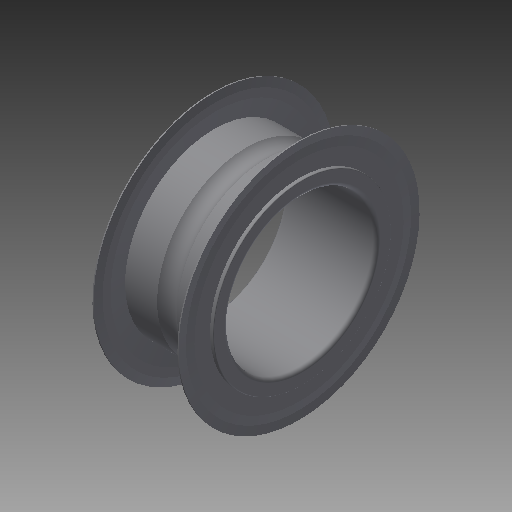
# Autodesk Inventor part: W 627/4-2Z_PART1
Saved by Autodesk Inventor 2018.3 (Build 223284000, 284)
## iProperties
Category: PARTsolutions
Company: SKF
Created: 2018-07-21
Part Number: W 627/4-2Z_PART1
Material: Generic
Catalog Web Link: www.cadenas.de
Description: -Deep groove ball bearings, stainless steel, single row
Vendor: SKF
Document SubType Name: Modeling
Designer: psadmin
Manufacturer: SKF
Mass: 0.0145905 g
Surface Area: 1.40149 cm^2
Volume: 0.0145905 cm^3
Density: 1 g/cm^3
Appearance: PSOLRGB-175-175-175
PSOL_IDENT_0: {$CADENAS_DATA\23d-libs\skf\bearings_units_and_housings\ball_bearings\deep_groove_ball_bearings\deep
PSOL_IDENT_1: _groove_ball_bearings_stainless_steel\bb1_004_104.prj},199 {VTYP=3D},{NB=W 627/4-2Z_PART1},{LINA=W 6
PSOL_IDENT_2: 27/4-2Z_PART1},{NN=BB1_004_104_PART1},{NOPRJ=TRUE},{DATE=13.07.2018 14:28:03},{GEOMDATE=26.07.2017 1
PSOL_IDENT_3: 2:34:56},{VERSION=},{LINEID=77220},{WBVAR=},{WBNUMERIC=}  {NB=W 627/4-2Z_PART1},{LINA=W 627/4-2Z_PAR
PSOL_IDENT_4: T1},{KT=DUMMY},{PRODUCTID=},{DESIGNATION=W 627/4-2Z},{DD=4.000},{D=7.000},{B=2.500},{DD1=4.800},{DD2=
PSOL_IDENT_5: MIN},{D1=6.000},{D2=6.500},{R12A=0.100},{LOAD1=0.143},{LOAD2=0.053},{LOAD3=0.002},{SPEED1=75000},{SP
PSOL_IDENT_6: EED2=},{MASS=0.000},{PITCH=5.400},{DW=0.800},{Z=11.000},{II=1.000},{TYPEID=MIN},{YALG=2.4},{HALG=0.4
PSOL_IDENT_7: },{HELP=0.5},{HELP2=0.25},{YALG1=3},{HALG1=0.5},{TAXONOMY=2},{DESIGN=dgbbw2z},{MAPPING=BCZ50,DESIGNA
PSOL_IDENT_8: TION|IRD01,DD|ORD10,D|BCW30,B|IRD30,DD1|ORD30,D1|ORD43,D2|IRD43,DD2|ORR20,R12A|BCC02,LOAD1|BCC16,LOA
PSOL_IDENT_9: D2|BCC12,LOAD3|BCC45,SPEED1|BCM01,MASS|BCD50,PITCH|RBD10,DW|BCN81,Z|BCN80,II},{DESIGNLIST=dgbbw2z,dg
PSOL_IDENT_10: bbw,dgbbw2rs},{SH=2.4},{SORT=DD},{RHELP=0.1},{PIM=W 627/4-2Z},{R12=0.1},{HIDE=MIN}
NT: Deep groove ball bearings, stainless steel, single row
NB: W 627/4-2Z_PART1
NBSYN: $DESIGNATION._PART1
LINA: W 627/4-2Z_PART1
SUPPLIER: SKF
ARTICLENO: W 627/4-2Z_PART1
BOMINFO: W 627/4-2Z_PART1
CREATOR: CADENAS GmbH
Title: W 627/4-2Z_PART1
Author: Cadenas PARTsolutions
Comments: Deep groove ball bearings, stainless steel, single row
Autodesk Inventor part; units mm, degrees
ref_plane "YZ Plane" through (0, 0, 0) normal (1, 0, 0) x (0, 1, 0)
ref_plane "XZ Plane" through (0, 0, 0) normal (0, 1, 0) x (-1, 0, 0)
ref_plane "XY Plane" through (0, 0, 0) normal (0, 0, 1) x (1, 0, 0)
sketch "Sketch_6" plane through (0, 0, 0) normal (0, 0, 1) x (1, 0, 0)
  line L0 (50, 0) -> (-50, 0)
  line L1 (0, 2.38) -> (0, 2.1)
  arc A0 (0, 2.1) -> (0.1, 2) centre (0.1, 2.1) ccw
  line L2 (0.1, 2) -> (2.4, 2)
  arc A1 (2.4, 2) -> (2.5, 2.1) centre (2.4, 2.1) ccw
  line L3 (2.5, 2.1) -> (2.5, 2.38)
  arc A2 (2.5, 2.38) -> (2.48, 2.4) centre (2.48, 2.38) ccw
  line L4 (2.48, 2.4) -> (1.5146, 2.4)
  arc A3 (0.9854, 2.4) -> (1.5146, 2.4) centre (1.25, 2.7) ccw
  line L5 (0.9854, 2.4) -> (0.02, 2.4)
  arc A4 (0.02, 2.4) -> (0, 2.38) centre (0.02, 2.38) ccw
  constraints: 12 end point, 10 point on circle, 5 centre point
revolve "Revolution1" add sketch "Sketch_6" angle 360 about axis through (50, 0, 0) along (1, 0, 0)
sketch "Sketch_11" plane through (0, 0, 0) normal (0, 0, 1) x (1, 0, 0)
  line L0 (50, 0) -> (-50, 0)
  line L1 (0.09, 3.25) -> (0.105, 3.035)
  line L2 (0.105, 3.035) -> (0.09, 2.82)
  line L3 (0.09, 2.82) -> (0.09, 2.39)
  line L4 (0.09, 2.39) -> (0.12, 2.39)
  line L5 (0.12, 2.39) -> (0.15, 2.82)
  line L6 (0.15, 2.82) -> (0.15, 3.035)
  line L7 (0.15, 3.035) -> (0.12, 3.25)
  line L8 (0.12, 3.25) -> (0.09, 3.25)
  constraints: 18 end point
revolve "Revolution2" add sketch "Sketch_11" angle 360 about axis through (50, 0, 0) along (1, 0, 0)
sketch "Sketch_12" plane through (0, 0, 0) normal (0, 0, 1) x (1, 0, 0)
  line L0 (50, 0) -> (-50, 0)
  line L1 (2.35, 3.035) -> (2.35, 2.82)
  line L2 (2.35, 2.82) -> (2.38, 2.39)
  line L3 (2.38, 2.39) -> (2.41, 2.39)
  line L4 (2.41, 2.39) -> (2.41, 2.82)
  line L5 (2.41, 2.82) -> (2.395, 3.035)
  line L6 (2.395, 3.035) -> (2.41, 3.25)
  line L7 (2.41, 3.25) -> (2.38, 3.25)
  line L8 (2.38, 3.25) -> (2.35, 3.035)
  constraints: 18 end point
revolve "Revolution3" add sketch "Sketch_12" angle 360 about axis through (50, 0, 0) along (1, 0, 0)
body "Solid1"
